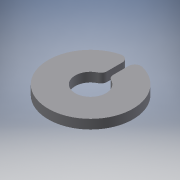
# Autodesk Inventor part: FrontTerm
Saved by Autodesk Inventor 2016 (Build 200138000, 138)
## iProperties
Created: 2015-04-23
Part Number: FrontTerm
Material: Generic
Document SubType Name: Modeling
Designer: JR
Density: 1 g/cm^3
Appearance: Default
Author: JR
Autodesk Inventor part; units mm, degrees
ref_plane "YZ Plane" through (0, 0, 0) normal (1, 0, 0) x (0, 1, 0)
ref_plane "XZ Plane" through (0, 0, 0) normal (0, 1, 0) x (-1, 0, 0)
ref_plane "XY Plane" through (0, 0, 0) normal (0, 0, 1) x (1, 0, 0)
sketch "Sketch1" plane through (0, 0, 0) normal (0, 0, 1) x (1, 0, 0)
  arc A0 (-3.5106, 13.2943) -> (3.5106, 13.2943) centre (0, 0) ccw
  circle A1 centre (0, 0) radius 4.5 construction
  line L0 (-1, 11.3606) -> (-1, 3.5)
  line L1 (1, 3.5) -> (1, 11.3606)
  arc A2 (-1, 3.5) -> (1, 3.5) centre (0, 3.5) ccw
  line L2 (-9.75, -9.75) -> (9.75, -9.75) construction
  line L3 (9.75, -9.75) -> (9.75, 9.75) construction
  line L4 (9.75, 9.75) -> (-9.75, 9.75) construction
  line L5 (-9.75, 9.75) -> (-9.75, -9.75) construction
  line L6 (-9.75, -9.75) -> (9.75, 9.75) construction
  line L7 (9.75, -9.75) -> (-9.75, 9.75) construction
  arc A3 (-1, 11.3606) -> (-3.5106, 13.2943) centre (-3, 11.3606) ccw
  arc A4 (3.5106, 13.2943) -> (1, 11.3606) centre (3, 11.3606) ccw
  point P0 (0, 6.1182)
  point P1 (0, 4.5)
  point P2 (0, 2.5)
  point P3 (0, 2.5)
  dimension "d1" = 9
  dimension "d0" = 27.5
  dimension "d2" = 2
  dimension "d3" = 2
  dimension "d5" = 19.5
  dimension "d9" = 19.5
  dimension "d10" = 2
  constraints: 16 end point, 9 point on circle, 6 tangent, 4 centre point, 4 midpoint, 4 vertical alignment, 3 coincident, 3 parallel, 1 equal radius, 1 horizontal, 1 perpendicular, 2 other
  measures "d0" diameter of A0
  measures "d2" diameter of A2
  measures "d3" distance of point (0, 4.5) point (0, 2.5)
  measures "d5" distance of L3.end L2.end
  measures "d9" distance of L3.end L4.end
  measures "d10" radius of A3
extrude "Extrusion1" add sketch "Sketch1" along normal blind 3
sketch "Sketch2" plane through (0, 0, 3) normal (0, 0, 1) x (1, 0, 0)
  circle A0 centre (0, 0) radius 5
  dimension "d11" = 10
  constraints: 1 centre point, 1 coincident
  measures "d11" diameter of A0
extrude "Extrusion2" cut sketch "Sketch2" against normal through all
fillet "Fillet1" radius 2 2 edges at (-1, 4.899, 1.5) (1, 4.899, 1.5)
body "Solid1"
